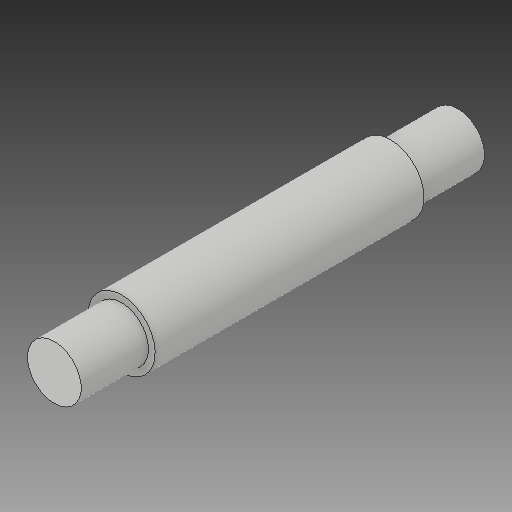
# Autodesk Inventor part: eixo
Saved by Autodesk Inventor 2019 (Build 230136000, 136)
## iProperties
Created: 2020-04-04
Part Number: eixo
Material: Generic
Document SubType Name: Modeling
Designer: Hermann
Density: 1 g/cm^3
Appearance: Default
Author: Hermann
Autodesk Inventor part; units mm, degrees
ref_plane "YZ Plane" through (0, 0, 0) normal (1, 0, 0) x (0, 1, 0)
ref_plane "XZ Plane" through (0, 0, 0) normal (0, 1, 0) x (-1, 0, 0)
ref_plane "XY Plane" through (0, 0, 0) normal (0, 0, 1) x (1, 0, 0)
sketch "Sketch1" plane through (0, 0, 0) normal (1, 0, 0) x (0, 1, 0)
  line L0 (0, 10) -> (4, 10)
  line L1 (4, 10) -> (4, 0)
  line L2 (4, 0) -> (5, 0)
  line L3 (5, 0) -> (5, -40)
  line L4 (5, -40) -> (4, -40)
  line L5 (4, -40) -> (4, -50)
  line L6 (4, -50) -> (0, -50)
  line L7 (0, -50) -> (0, 10)
  point P0 (0, 0)
  dimension "d0" = 4
  dimension "d1" = 10
  dimension "d2" = 10
  dimension "d3" = 5
  dimension "d4" = 0
  dimension "d5" = 0
  dimension "d6" = 40
  constraints: 16 end point, 6 perpendicular, 2 point on line, 1 horizontal
  measures "d0" distance between parallel lines of L7 L5
  measures "d1" distance between parallel lines of L0 L2
  measures "d2" distance between parallel lines of L4 L6
  measures "d3" distance between parallel lines of L7 L3
  measures "d4" distance from line of L2 point (0, 0)
  measures "d5" distance from line of point (0, 0) L7
  measures "d6" distance from line of L2.end L4
revolve "Revolution1" add sketch "Sketch1" angle 360 about axis through (0, 0, -50) along (0, 0, 1)
body "Solid1"
